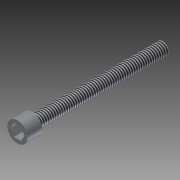
# Autodesk Inventor part: Bolt 8-32 bracket BD Drill motor mount
Saved by Autodesk Inventor 2012 (Build 160160000, 160)
## iProperties
Created: 2012-06-30
Part Number: Bolt 8-32 bracket BD Drill motor mount
Material: Default
Document SubType Name: Modeling
Designer: Bruce
Density: 1 g/cm^3
Author: Bruce
Autodesk Inventor part; units mm, degrees
ref_plane "YZ Plane" through (0, 0, 0) normal (1, 0, 0) x (0, 1, 0)
ref_plane "XZ Plane" through (0, 0, 0) normal (0, 1, 0) x (-1, 0, 0)
ref_plane "XY Plane" through (0, 0, 0) normal (0, 0, 1) x (1, 0, 0)
sketch "Sketch1" plane through (0, 0, 0) normal (0, 0, 1) x (1, 0, 0)
  circle A0 centre (0, 0) radius 3.429
  circle A1 centre (0, 0) radius 2.0828
  line L0 (1.2025, 2.0828) -> (2.405, 0)
  line L1 (2.405, 0) -> (1.2025, -2.0828)
  line L2 (1.2025, -2.0828) -> (-1.2025, -2.0828)
  line L3 (-1.2025, -2.0828) -> (-2.405, 0)
  line L4 (-2.405, 0) -> (-1.2025, 2.0828)
  line L5 (-1.2025, 2.0828) -> (1.2025, 2.0828)
  dimension "d0" = 4.1656
  dimension "d1" = 6.858
  constraints: 12 end point, 3 coincident, 2 centre point, 1 horizontal, 1 tangent, 13 other
  measures "d0" diameter of A1
  measures "d1" diameter of A0
extrude "Extrusion1" add sketch "Sketch1" against normal blind 44.45 contours A1
extrude "Extrusion2" add sketch "Sketch1" along normal blind 5.08
thread "Thread1" size "8-32 UNC" class "2A" standard "ANSI Unified Screw Threads" full length
body "Solid1"
